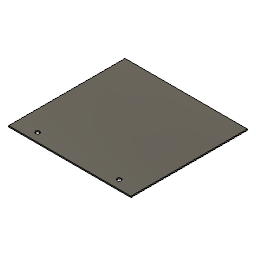
Abdeckplatte (Autodesk Fusion 360 design; units mm, degrees)
part number: 2025-12-10-18-01-09-044
Autodesk Fusion 360 part; units mm, degrees
note: some values were not read from the file. Set by a fixed rule: which sketch regions a step uses.
sketch "Skizze1" plane through (0, 0, 0) normal (0, 0, 1) x (1, 0, 0)
  line L0 (0, 0) -> (210, 0)
  line L1 (210, 0) -> (210, 200)
  line L2 (210, 200) -> (0, 200)
  line L3 (0, 200) -> (0, 0)
  line L4 (0, 0) -> (210, 0)
  line L5 (210, 0) -> (210, 30)
  line L6 (210, 30) -> (0, 30)
  line L7 (0, 30) -> (0, 0)
  line L8 (0, 15) -> (210, 15) construction
  line L9 (0, 15) -> (35, 15)
  circle A0 centre (35, 15) radius 3.5
  line L10 (210, 15) -> (175, 15)
  circle A1 centre (175, 15) radius 3.5
  dimension "d1" = 210
  dimension "d2" = 200
  dimension "d3" = 7
  dimension "d4" = 7
  constraint horizontal L0
  constraint vertical L1
  constraint horizontal L2
  constraint vertical L3
  constraint coincident L0.start L3.end
  constraint horizontal L4
  constraint vertical L5
  constraint horizontal L6
  constraint vertical L7
  constraint coincident L1 L5.end
  constraint midpoint L7 L8.start
  constraint midpoint L5 L8.end
  constraint coincident L8 L9.end
  constraint coincident L9.end A0.centre
  constraint coincident L8 L10.end
  constraint coincident L10.end A1.centre
  measures "d1" distance of L0.start L0.end
  measures "d2" distance of L0.start L2.end
  measures "d3" diameter of A0
  measures "d4" diameter of A1
extrude "Extrusion1" add sketch "Skizze1" along normal blind 2
